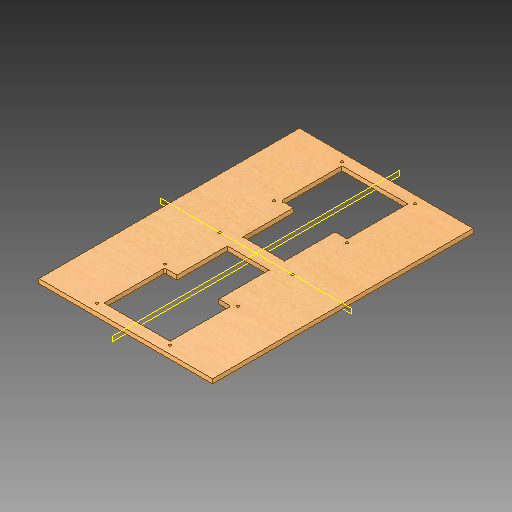
# Autodesk Inventor part: socle-robot
Saved by Autodesk Inventor 2019 (Build 230136000, 136)
## iProperties
Created: 2018-04-01
Part Number: socle-robot
Material: Générique
Document SubType Name: Modeling
Designer: franc
Density: 1 g/cm^3
Appearance: Pin jaune - Massif moiré clair faible lustre
Mass: 218.624 g
Surface Area: 969.836 cm^2
Volume: 218.624 cm^3
Author: franc
Autodesk Inventor part; units mm, degrees
ref_plane "YZ Plane" through (0, 0, 0) normal (1, 0, 0) x (0, 1, 0)
ref_plane "XZ Plane" through (0, 0, 0) normal (0, 1, 0) x (-1, 0, 0)
ref_plane "XY Plane" through (0, 0, 0) normal (0, 0, 1) x (1, 0, 0)
sketch "Esquisse1" plane through (0, 0, 0) normal (0, 1, 0) x (-1, 0, 0)
  line L0 (81.9588, 98.0854) -> (-118.0412, 98.0854)
  line L1 (-118.0412, 98.0854) -> (-118.0412, -201.9146)
  line L2 (-118.0412, -201.9146) -> (81.9588, -201.9146)
  line L3 (81.9588, -201.9146) -> (81.9588, 98.0854)
  point P0 (0, 0)
  dimension "d0" = 300
  dimension "d1" = 200
  constraints: 8 end point, 2 parallel, 1 horizontal, 1 perpendicular
  measures "d0" distance of L2.end L0.start
  measures "d1" distance of L0.start L0.end
extrude "Extrusion1" add sketch "Esquisse1" along normal blind 5
sketch "Esquisse2" plane through (0, 5, 0) normal (0, 1, 0) x (1, 0, 0)
  circle A0 centre (43.0412, 167.9146) radius 2.5 projected
  arc A1 (33.0412, 150.9146) -> (35.0412, 152.9146) centre (33.0412, 152.9146) ccw projected
  line L0 (33.0412, 150.9146) -> (3.0412, 150.9146) projected
  arc A2 (1.0412, 152.9146) -> (3.0412, 150.9146) centre (3.0412, 152.9146) ccw projected
  line L1 (1.0412, 152.9146) -> (1.0412, 186.9146) projected
  arc A3 (3.0412, 188.9146) -> (1.0412, 186.9146) centre (3.0412, 186.9146) ccw projected
  line L2 (3.0412, 188.9146) -> (33.0412, 188.9146) projected
  arc A4 (35.0412, 186.9146) -> (33.0412, 188.9146) centre (33.0412, 186.9146) ccw projected
  line L3 (35.0412, 186.9146) -> (35.0412, 152.9146) projected
  circle A5 centre (-6.9588, 167.9146) radius 2.5 projected
  circle A6 centre (48.0412, 172.9146) radius 1 projected
  circle A7 centre (38.0412, 172.9146) radius 1 projected
  circle A8 centre (-11.9588, 172.9146) radius 1 projected
  circle A9 centre (-11.9588, 162.9146) radius 1 projected
  circle A10 centre (-1.9588, 162.9146) radius 1 projected
  circle A11 centre (-1.9588, 172.9146) radius 1 projected
  circle A12 centre (38.0412, 162.9146) radius 1 projected
  circle A13 centre (48.0412, 162.9146) radius 1 projected
  circle A14 centre (60.0412, 114.9146) radius 1.5 projected
  circle A15 centre (-23.9588, 192.9146) radius 1.5 projected
  circle A16 centre (60.0412, 192.9146) radius 1.5 projected
  circle A17 centre (-23.9588, 114.9146) radius 1.5 projected
  circle A18 centre (-23.9588, 51.9146) radius 1.5 projected
  circle A19 centre (60.0412, -11.0854) radius 1.5 projected
  circle A20 centre (-23.9588, -89.0854) radius 1.5 projected
  circle A21 centre (60.0412, -89.0854) radius 1.5 projected
  circle A22 centre (-23.9588, -11.0854) radius 1.5 projected
  circle A23 centre (60.0412, 51.9146) radius 1.5 projected
  circle A24 centre (43.0412, -64.0854) radius 2.5 projected
  circle A25 centre (48.0412, -59.0854) radius 1 projected
  circle A26 centre (38.0412, -59.0854) radius 1 projected
  circle A27 centre (-1.9588, -69.0854) radius 1 projected
  circle A28 centre (-1.9588, -59.0854) radius 1 projected
  circle A29 centre (-11.9588, -59.0854) radius 1 projected
  circle A30 centre (-11.9588, -69.0854) radius 1 projected
  circle A31 centre (38.0412, -69.0854) radius 1 projected
  circle A32 centre (48.0412, -69.0854) radius 1 projected
  circle A33 centre (-6.9588, -64.0854) radius 2.5 projected
  arc A34 (1.0412, -83.0854) -> (3.0412, -85.0854) centre (3.0412, -83.0854) ccw projected
  line L4 (1.0412, -83.0854) -> (1.0412, -49.0854) projected
  arc A35 (3.0412, -47.0854) -> (1.0412, -49.0854) centre (3.0412, -49.0854) ccw projected
  line L5 (3.0412, -47.0854) -> (33.0412, -47.0854) projected
  arc A36 (35.0412, -49.0854) -> (33.0412, -47.0854) centre (33.0412, -49.0854) ccw projected
  line L6 (35.0412, -49.0854) -> (35.0412, -83.0854) projected
  arc A37 (33.0412, -85.0854) -> (35.0412, -83.0854) centre (33.0412, -83.0854) ccw projected
  line L7 (33.0412, -85.0854) -> (3.0412, -85.0854) projected
  arc A38 (-19.9588, 120.9146) -> (-17.9588, 118.9146) centre (-17.9588, 120.9146) ccw projected
  line L8 (-19.9588, 120.9146) -> (-19.9588, 146.9146) projected
  arc A39 (-17.9588, 148.9146) -> (-19.9588, 146.9146) centre (-17.9588, 146.9146) ccw projected
  line L9 (-17.9588, 148.9146) -> (54.0412, 148.9146) projected
  arc A40 (56.0412, 146.9146) -> (54.0412, 148.9146) centre (54.0412, 146.9146) ccw projected
  line L10 (56.0412, 146.9146) -> (56.0412, 120.9146) projected
  arc A41 (54.0412, 118.9146) -> (56.0412, 120.9146) centre (54.0412, 120.9146) ccw projected
  line L11 (54.0412, 118.9146) -> (-17.9588, 118.9146) projected
  arc A42 (54.0412, -45.0854) -> (56.0412, -43.0854) centre (54.0412, -43.0854) ccw projected
  line L12 (54.0412, -45.0854) -> (-17.9588, -45.0854) projected
  arc A43 (-19.9588, -43.0854) -> (-17.9588, -45.0854) centre (-17.9588, -43.0854) ccw projected
  line L13 (-19.9588, -43.0854) -> (-19.9588, -17.0854) projected
  arc A44 (-17.9588, -15.0854) -> (-19.9588, -17.0854) centre (-17.9588, -17.0854) ccw projected
  line L14 (-17.9588, -15.0854) -> (54.0412, -15.0854) projected
  arc A45 (56.0412, -17.0854) -> (54.0412, -15.0854) centre (54.0412, -17.0854) ccw projected
  line L15 (56.0412, -17.0854) -> (56.0412, -43.0854) projected
  line L16 (-27.9588, -93.0854) -> (64.0412, -93.0854) projected
  line L17 (64.0412, -93.0854) -> (64.0412, 196.9146) projected
  line L18 (64.0412, 196.9146) -> (-27.9588, 196.9146) projected
  line L19 (-27.9588, 196.9146) -> (-27.9588, -93.0854) projected
  line L20 (-5.9588, -15.0854) -> (42.0412, -15.0854)
  line L21 (42.0412, -15.0854) -> (42.0412, 42.9146)
  line L22 (42.0412, 42.9146) -> (-5.9588, 42.9146)
  line L23 (-5.9588, 42.9146) -> (-5.9588, -15.0854)
  line L24 (-19.9588, -43.0854) -> (56.0412, -43.0854)
  line L25 (56.0412, -43.0854) -> (56.0412, -85.0854)
  line L26 (56.0412, -85.0854) -> (-19.9588, -85.0854)
  line L27 (-19.9588, -85.0854) -> (-19.9588, -43.0854)
  line L28 (-19.9588, 146.9146) -> (56.0412, 146.9146)
  line L29 (56.0412, 146.9146) -> (56.0412, 188.9146)
  line L30 (56.0412, 188.9146) -> (-19.9588, 188.9146)
  line L31 (-19.9588, 188.9146) -> (-19.9588, 146.9146)
  line L32 (-5.9588, 118.9146) -> (42.0412, 118.9146)
  line L33 (42.0412, 118.9146) -> (42.0412, 60.9146)
  line L34 (42.0412, 60.9146) -> (-5.9588, 60.9146)
  line L35 (-5.9588, 60.9146) -> (-5.9588, 118.9146)
  dimension "d7" = 14
  dimension "d8" = 14
  dimension "d9" = 58
  dimension "d10" = 0
  dimension "d11" = 0
  dimension "d14" = 14
  dimension "d15" = 14
  dimension "d16" = 58
  constraints: 32 end point, 8 parallel, 4 horizontal, 4 perpendicular, 3 point on line
  measures "d7" distance between parallel lines of L23 L13
  measures "d8" distance between parallel lines of L21 L15
  measures "d9" distance between parallel lines of L22 L14
  measures "d10" distance between parallel lines of L7 L26
  measures "d11" distance between parallel lines of L30 L2
  measures "d14" distance between parallel lines of L8 L35
  measures "d15" distance between parallel lines of L10 L33
  measures "d16" distance between parallel lines of L32 L34
extrude "Extrusion2" cut sketch "Esquisse2" against normal through all contours A0 | L0 A2 L1 A3 L2 A4 L3 A1 | A1 L3 A4 L30 L29 A40 L9 A39 L31 A3 L1 A2 L0 | L28 A39 L9 A40 | L10 A41 L11 A38 L8 L28 | L33 L34 L35 L11 | A5 | A6 | A7 | A8 | A9 | A10 | A11 | A12 | A13 | A14 | A15 | A16 | A17 | A18 | A19 | A20 | A21 | A22 | A23 | A24 | A25 | A26 | A27 | A28 | A29 | A30 | A31 | A32 | A33 | L4 A35 L5 A36 L6 A37 L7 A34 | A34 L26 L27 A43 L12 A42 L25 A37 L6 A36 L5 A35 L4 | L24 A42 L12 A43 | L13 A44 L14 A45 L15 L24 | L23 L22 L21 L14
ref_plane "Plan de construction1" through (-81.9588, 0, -51.9146) normal (0, 0, 1) x (1, 0, 0)
ref_plane "Plan de construction2" through (18.0412, 0, 98.0854) normal (1, 0, 0) x (0, 0, -1)
